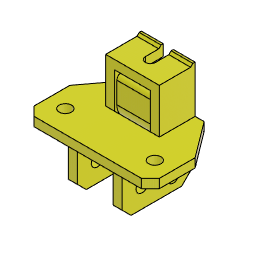
Idler Buddy Front_1x (Autodesk Fusion 360 design; units mm, degrees)
Autodesk Fusion 360 part; units mm, degrees
ref_plane "WorkPlane1" through (170, 280, 322.55) normal (0, -1, 0) x (0, 0, 1)
sketch "Sketch1" plane through (170, 280, 322.55) normal (0, -1, 0) x (1, 0, 0)
  line L0 (0, 4) -> (56, 4)
  line L1 (56, 4) -> (56, 0)
  line L2 (56, 0) -> (0, 0)
  line L3 (0, 0) -> (0, 4)
  dimension "d6344" = 56
  dimension "d6345" = 4
  constraint horizontal L0
  constraint vertical L1
  constraint horizontal L2
  constraint vertical L3
  constraint coincident L2.end L3.start
  measures "d6344" distance of L0.start L0.end
  measures "d6345" distance of L0.start L2.end
extrude "Extrude2" add sketch "Sketch1" against normal blind 20 makes body 1
ref_plane "WorkPlane2" through (198, 290, 324.55) normal (-1, 0, 0) x (0, 0, 1)
sketch "Sketch2" plane through (198, 290, 324.55) normal (-1, 0, 0) x (0, 1, 0)
  line L0 (-10, -2) -> (-10, 2)
  line L1 (-10, 2) -> (10, 2)
  line L2 (10, -2) -> (10, 2)
  line L3 (-10, -2) -> (10, -2)
  circle A0 centre (2.35, 13) radius 2.75
  circle A1 centre (2.35, 13) radius 9 construction
  circle A2 centre (2.35, 13) radius 6 construction
  circle A3 centre (16.25, 16.75) radius 2.25
  line L4 (10, -2) -> (26, -2) construction
  line L5 (26, -2) -> (26, 22)
  line L6 (-10, 22) -> (26, 22)
  line L7 (10, -2) -> (10, -22)
  line L8 (10, -22) -> (26, -22)
  line L9 (26, -22) -> (26, -2)
  circle A4 centre (18, -39.5) radius 2.5
  circle A5 centre (18, -39.5) radius 4.5
  circle A6 centre (18, -39.5) radius 7.5
  line L10 (22.5, -39.5) -> (22.5, -32)
  line L11 (13.5, -32) -> (13.5, -39.5)
  line L12 (20.5, -39.5) -> (20.5, -32)
  line L13 (10.5, -39.5) -> (10.5, -51)
  line L14 (10.5, -51) -> (25.5, -51)
  line L15 (25.5, -51) -> (25.5, -32)
  line L16 (18, -39.5) -> (18, -51) construction
  arc A7 (18, -35) -> (20.5, -32.5) centre (18, -32.5) ccw
  line L17 (18, -22) -> (18, 22) construction
  circle A8 centre (16.25, 16.75) radius 4.25
  line L18 (20.5, -32.5) -> (20.5, 22) construction
  line L19 (2.35, 13) -> (16.25, 16.75) construction
  line L20 (-10, -2) -> (-10, 22)
  line L21 (13.5, -32) -> (25.5, -32)
  line L22 (-6.65, 22) -> (-6.65, 2)
  point P0 (-10, -2)
  point P1 (16.25, 16.75)
  point P2 (18, -22)
  dimension "d6354" = 5.5
  dimension "d6360" = 18
  dimension "d6361" = 12
  dimension "d62" = 4.5
  dimension "d110" = 2
  dimension "d113" = 5
  dimension "d114" = 2
  dimension "d115" = 10
  dimension "d116" = 3
  dimension "d117" = 16
  dimension "d118" = 4
  dimension "d120" = 2.5
  dimension "d121" = 16
  dimension "d122" = 20
  dimension "d131" = 10.5
  dimension "d132" = 2
  dimension "d189" = 6.35
  dimension "d199" = 10
  dimension "d216" = 3
  constraint concentric A0 A1
  constraint concentric A1 A2
  constraint coincident P1 A3.centre
  constraint coincident L2.start L3.end
  constraint perpendicular L2 L4
  constraint perpendicular L3 L5
  constraint coincident L5.end L6.end
  constraint tangent A1 L6
  constraint perpendicular L4 L7
  constraint perpendicular L7 L8
  constraint perpendicular L8 L9
  constraint coincident L4.end L5.start
  constraint concentric A4 A5
  constraint concentric A5 A6
  constraint coincident A5 L10.start
  constraint tangent A5 L10
  constraint vertical L10
  constraint coincident A5 L11.end
  constraint tangent A5 L11
  constraint coincident A4 L12.start
  constraint tangent A4 L12
  constraint perpendicular L4 L12
  constraint coincident A6 L13.start
  constraint tangent A6 L13
  constraint parallel L11 L13
  constraint perpendicular L13 L14
  constraint perpendicular L14 L15
  constraint tangent A6 L15
  constraint coincident A4.centre A5.centre
  constraint parallel L15 L16
  constraint midpoint L14 L16.end
  constraint coincident A5 A7.start
  constraint tangent A5 A7
  constraint tangent L12 A7
  constraint midpoint L8 P2
  constraint vertical L16.end P2
  constraint coincident P2 L17.start
  constraint coincident L6 L17.end
  constraint perpendicular L6 L17
  constraint concentric A3 A8
  constraint tangent A7 L18
  constraint tangent A8 L18
  constraint coincident L6 L18.end
  constraint coincident A0.centre A1.centre
  constraint coincident P0 L0.start
  constraint coincident L6 L20.end
  constraint coincident L6.start L20.end
  constraint horizontal L6
  constraint vertical L11
  constraint perpendicular L18 L21
  constraint coincident L15.end L21.end
  constraint coincident L10.end L21
  constraint tangent A6 L21
  constraint horizontal L21
  constraint coincident L21 L12.end
  constraint perpendicular L6 L20
  constraint coincident L6 L22.start
  constraint coincident L1 L22.end
  constraint perpendicular L1 L22
  constraint tangent A1 L22
  measures "d6354" diameter of A0
  measures "d6360" diameter of A1
  measures "d6361" diameter of A2
  measures "d62" diameter of A3
  measures "d110" distance of L1 A1
  measures "d113" diameter of A4
  measures "d114" distance of A4 A5
  measures "d116" distance of A5 A6
  measures "d118" distance of A6 L14
  measures "d120" radius of A7
  measures "d121" distance of L7.end L8.end
  measures "d122" distance of L2.start L7.end
  measures "d132" distance of A3 A8
  measures "d189" distance of A2 L20
  measures "d199" vertical distance of L8.end L15.end
  measures "d216" distance of A3 L6
extrude "Extrude3" add sketch "Sketch2" along normal blind 4 from surface at 8 contours L0 L1 L2 L3 L20 | L1 L2 L5 L6 L7 L8 L9 L22 | A8 bodies 1
hole "Hole6" at (178, 290, 326.55) direction (0, 0, -1) diameter 5.5 depth 17 tip angle 118 bodies 1
mirror "Mirror1" about plane through (198, 290, 324.55) normal (-1, 0, 0) of "Extrude3", "Hole6"
sketch "Sketch19" plane through (0, 316, 0) normal (0, 1, 0) x (-1, 0, 0)
  line L0 (-190, 346.55) -> (-190, 302.55)
  line L1 (-190, 302.55) -> (-186, 302.55)
  line L2 (-186, 302.55) -> (-186, 346.55)
  line L3 (-186, 346.55) -> (-190, 346.55)
  line L4 (-206, 326.55) -> (-206, 346.55)
  line L5 (-206, 346.55) -> (-210, 346.55)
  line L6 (-210, 326.55) -> (-210, 346.55)
  line L7 (-226, 326.55) -> (-226, 322.55)
  line L8 (-170, 326.55) -> (-186, 326.55)
  line L9 (-190, 326.55) -> (-206, 326.55)
  line L10 (-210, 326.55) -> (-226, 326.55)
  line L11 (-170, 322.55) -> (-170, 326.55)
  line L12 (-186, 326.55) -> (-186, 346.55)
  line L13 (-190, 346.55) -> (-186, 346.55)
  line L14 (-190, 326.55) -> (-190, 346.55)
  line L15 (-210, 346.55) -> (-186, 346.55)
  line L16 (-210, 342.55) -> (-186, 342.55)
  line L17 (-210, 326.55) -> (-210, 322.55)
  line L18 (-210, 346.55) -> (-186, 346.55)
  line L19 (-186, 346.55) -> (-186, 347.55)
  line L20 (-186, 347.55) -> (-210, 347.55)
  line L21 (-210, 347.55) -> (-210, 346.55)
  line L22 (-206, 302.55) -> (-206, 322.55)
  line L23 (-206, 302.55) -> (-210, 302.55)
  line L24 (-210, 302.55) -> (-210, 322.55)
  line L25 (-226, 322.55) -> (-210, 322.55)
  line L26 (-206, 322.55) -> (-190, 322.55)
  line L27 (-186, 322.55) -> (-170, 322.55)
  line L28 (-186, 302.55) -> (-186, 322.55)
  line L29 (-190, 302.55) -> (-190, 322.55)
  line L30 (-190, 302.55) -> (-186, 302.55)
  line L31 (-186, 326.55) -> (-186, 322.55)
  dimension "d124" = 4
  dimension "d133" = 1
  constraint coincident L5.end L6.end
  constraint coincident L2.end L3.start
  constraint coincident L6 L16.start
  constraint perpendicular L12 L16
  constraint coincident L2 L16.end
  constraint coincident L6.start L10.start
  constraint horizontal L18
  constraint vertical L19
  constraint horizontal L20
  constraint vertical L21
  constraint coincident L17.end L24.end
  constraint coincident L8.end L12.start
  constraint coincident L27.start L28.end
  measures "d124" distance of L2.end L16.end
  measures "d133" distance of L2.end L19.end
extrude "Extrude29" add sketch "Sketch19" against normal blind 16 contours L0 L4 L14 L15 L16 L18 bodies 1
extrude "Extrude34" add 2 faces at (175.3333, 300, 323.8833) (215.3333, 300, 325.2167) along direction (0, 1, 0) blind 16 on bodies 1 bodies 1
chamfer "Chamfer11" distance 12 distance2 16 2 edges at (170, 316, 324.55) (226, 316, 324.55) measured on face at (188.6667, 316, 322.55) measured on face at (188.6667, 316, 322.55) on bodies 1
extrude "Extrude31" add sketch "Sketch19" against normal blind 1 contours L3 L5 L13 L15 L18 L19 L20 L21 bodies 1
chamfer "Chamfer12" distance 1 angle 45 1 edges at (198, 315, 346.55) on bodies 1
sketch "Sketch20" plane through (0, 0, 346.55) normal (0, 0, 1) x (-1, 0, 0)
  line L0 (-186, -300) -> (-210, -300)
  line L1 (-210, -300) -> (-210, -314)
  line L2 (-186, -314) -> (-186, -300)
  line L3 (-198, -300) -> (-198, -316) construction
  line L4 (-200.25, -308) -> (-200.25, -316)
  arc A0 (-200.25, -316) -> (-195.75, -316) centre (-198, -316) ccw
  line L5 (-195.75, -316) -> (-195.75, -308)
  arc A1 (-195.75, -308) -> (-200.25, -308) centre (-198, -308) ccw
  line L6 (-198, -308) -> (-198, -316) construction
  line L7 (-210, -314) -> (-186, -314)
  line L8 (-186, -316) -> (-210, -316)
  dimension "d128" = 4.5
  constraint midpoint L0 L3.start
  constraint tangent L4 A0
  constraint tangent A0 L5
  constraint parallel L4 L5
  constraint tangent L5 A1
  constraint tangent L4 A1
  constraint coincident L3.end A0.centre
  constraint midpoint L3 A1.centre
  constraint midpoint L3.end L8
  measures "d128" diameter of A0
extrude "Extrude30" cut sketch "Sketch20" along normal mid plane 12 contours L4 L5 A1 L7 | L4 L5 L7 L8 | A0 L8 bodies 1
chamfer "Chamfer9" distance 4 angle 45 2 edges at (226, 280, 324.55) (170, 280, 324.55) on bodies 1
chamfer "Chamfer13" distance 6 angle 45 2 edges at (188, 316, 302.55) (208, 316, 302.55) on bodies 1
chamfer "Chamfer14" distance 4 angle 45 2 edges at (208, 283.35, 302.55) (188, 283.35, 302.55) on bodies 1
copy_body "Body->Comp5" bodies 1 removing the originals makes body 2 in component "11mm Z Belt Buddy Front_1x"
extrude "Extrude32" add sketch "Sketch2" along normal blind 3.5 separate body contours A4 | A5 | A5 L12 A7 | A5 A6 L11 L12 A7 | A5 A6 L10 L11 | A5 A6 L10 L12 | A6 L11 L21 | A6 L10 L12 L21 | A6 L12 L21 | A6 L10 L15 L21 | A6 L13 L14 L15 makes body 3
extrude "Extrude33" add sketch "Sketch2" against normal blind 11.5 contours A4 | A5 A6 L11 L12 A7 | A5 A6 L10 L11 | A6 L11 L21 | A6 L12 L21 | A6 L10 L15 L21 | A6 L13 L14 L15 bodies 3
copy_body "Body->Comp6" bodies 3 removing the originals makes body 4 in component "11mm Z Belt Tension Buddy_1x"
sketch "Sketch1 (2)" plane through (209.5, 0, 0) normal (1, 0, 0) x (0, 1, 0) in component "11mm Z Belt Tension Buddy_1x"
  line L0 (315.5, 356.55) -> (315.5, 375.55)
  line L1 (315.5, 375.55) -> (300.5, 375.55)
  line L2 (300.5, 375.55) -> (300.5, 364.05)
  arc A0 (300.5, 364.05) -> (303.5, 358.05) centre (308, 364.05) ccw
  line L3 (303.5, 358.05) -> (303.5, 356.55)
  line L4 (308, 375.55) -> (308, 373.55) construction
  line L5 (304.5, 373.55) -> (311.5, 373.55)
  line L6 (311.5, 373.55) -> (311.5, 356.55)
  line L7 (311.5, 370.05) -> (304.5, 370.05)
  line L8 (304.5, 356.55) -> (304.5, 373.55)
  line L9 (305.75, 373.55) -> (305.75, 375.55)
  line L10 (310.25, 373.55) -> (310.25, 375.55)
  line L11 (312.5, 364.05) -> (312.5, 356.55)
  line L12 (303.5, 356.55) -> (310.5, 356.55)
  line L13 (310.5, 356.55) -> (310.5, 357.05)
  arc A1 (310.5, 357.05) -> (308, 359.55) centre (308, 357.05) ccw
  arc A2 (312.5, 364.05) -> (308, 359.55) centre (308, 364.05) ccw
  line L14 (312.5, 356.55) -> (315.5, 356.55)
  dimension "d142" = 7
  dimension "d143" = 3.5
  dimension "d144" = 2
  dimension "d145" = 4.5
  constraint midpoint L1 L4.start
  constraint perpendicular L1 L4
  constraint horizontal L5
  constraint vertical L6
  constraint horizontal L7
  constraint vertical L8
  constraint midpoint L4.end L5
  constraint coincident L5 L9.start
  constraint coincident L1 L9.end
  constraint perpendicular L1 L9
  constraint coincident L5 L10.start
  constraint coincident L1 L10.end
  constraint perpendicular L1 L10
  constraint symmetric L4 L9.end L10.end
  constraint coincident L6.end L12
  constraint coincident L7.start L6
  constraint coincident L8.start L12
  constraint coincident L7.end L8
  measures "d142" distance of L5.start L5.end
  measures "d143" distance of L5.start L7.end
  measures "d144" distance of L4.start L4.end
  measures "d145" distance of L9.end L10.end
hole "Hole1" at (202, 308, 375.55) direction (0, 0, -1) diameter 4.5 depth 5 tip angle 180 bodies 4 in component "11mm Z Belt Tension Buddy_1x"
extrude "Extrude1" cut sketch "Sketch1 (2)" against normal blind 16.5 contours L5 L6 L7 L8 bodies 4 in component "11mm Z Belt Tension Buddy_1x"
extrude "Extrude2'" cut sketch "Sketch1 (2)" against normal blind 7.5 contours L1 L5 L9 L10 bodies 4 in component "11mm Z Belt Tension Buddy_1x"
extrude "Extrude20" add sketch "Sketch2" along normal mid plane 15 separate body contours A8 makes body 5
fillet "Fillet1" radius 2 2 edges at (202, 300.5, 375.55) (202, 315.5, 375.55) on bodies 4 in component "11mm Z Belt Tension Buddy_1x"
copy_body "Body->Comp4" bodies 5 removing the originals makes body 6 in component "11mm Z Belt Buddy Front Spacer_1x"
component "11mm Z Belt Buddy Front_1x" placed x (1, 0, 0) y (0, 1, 0) z (0, 0, 1) at (0, 0, 0)
component "11mm Z Belt Tension Buddy_1x" placed x (1, 0, 0) y (0, 1, 0) z (0, 0, 1) at (-4, 0, -35)
component "11mm Z Belt Buddy Front Spacer_1x" placed x (1, 0, 0) y (0, 1, 0) z (0, 0, 1) at (0, 0, 0)
equation "d6363 = ( 12 / 2 ) * 1 mm + 2 mm"
equation "d7386 = 11 mm + 4 mm"
equation "d140 = -7.5 mm - 4 mm"
equation "d189 = 5.6 mm + 0.75 mm"
named bodies: "Idler Buddy Front_1x", "Belt Run", "11mm Z Belt Buddy Front Spacer_1x", "11mm Z Belt Buddy Front_1x", "11mm Z Belt Tension Buddy_1x"
